# Autodesk Inventor part: ADS1256IDBT
Saved by Autodesk Inventor 2016 (Build 200138000, 138)
## iProperties
Created: 2016-04-08
Part Number: ADS1256IDBT
Material: Generic
Document SubType Name: Modeling
Designer: Paschalis
Density: 1 g/cm^3
Appearance: SOP65P780X200-28N, ADS1256IDBT
Author: Paschalis
Autodesk Inventor part; units mm, degrees
ref_plane "YZ Plane" through (0, 0, 0) normal (1, 0, 0) x (0, 1, 0)
ref_plane "XZ Plane" through (0, 0, 0) normal (0, 1, 0) x (-1, 0, 0)
ref_plane "XY Plane" through (0, 0, 0) normal (0, 0, 1) x (1, 0, 0)
sketch "SOP65P780X200-28N, ADS1256IDBT_5" plane through (0, 0, 0) normal (0, 0, 1) x (1, 0, 0)
  line L0 (-4.0894, 5.334) -> (4.0894, 5.334)
  line L1 (4.0894, 5.334) -> (4.0894, -5.2578)
  line L2 (4.0894, -5.2578) -> (-4.0894, -5.2578)
  line L3 (-4.0894, -5.2578) -> (-4.0894, 5.334)
  constraints: 8 end point
extrude "Extrusion1" add sketch "SOP65P780X200-28N, ADS1256IDBT_5" along normal blind 1
body "Solid1"
